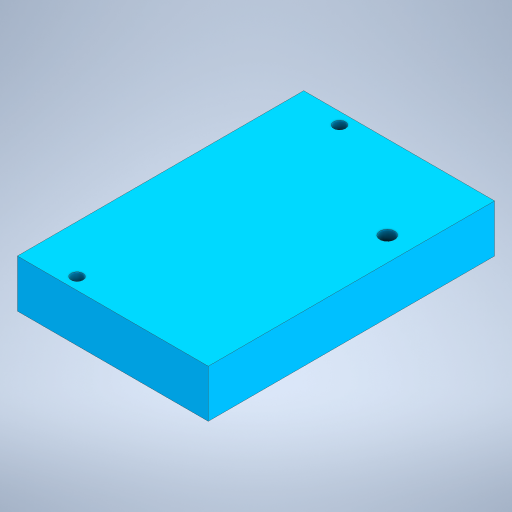
# Autodesk Inventor part: Top Plate for Side to Side motion
Saved by Autodesk Inventor 2023.1 (Build 271208000, 208)
## iProperties
Created: 2022-12-21
Part Number: Top Plate for Side to Side motion
Material: Generic
Document SubType Name: Modeling
Designer: shubh
Density: 1 g/cm^3
Appearance: Default
Author: shubh
Autodesk Inventor part; units mm, degrees
ref_plane "YZ Plane" through (0, 0, 0) normal (1, 0, 0) x (0, 1, 0)
ref_plane "XZ Plane" through (0, 0, 0) normal (0, 1, 0) x (-1, 0, 0)
ref_plane "XY Plane" through (0, 0, 0) normal (0, 0, 1) x (1, 0, 0)
sketch "Sketch1" plane through (0, 0, 0) normal (0, 1, 0) x (-1, 0, 0)
  line L0 (38.1, 76.2) -> (-63.5, 76.2)
  line L1 (-63.5, 76.2) -> (-63.5, -76.2)
  line L2 (-63.5, -76.2) -> (38.1, -76.2)
  line L3 (38.1, -76.2) -> (38.1, 76.2)
  circle A0 centre (-50.8, -31.75) radius 3.9751
  circle A1 centre (12.7, 69.85) radius 3.175
  circle A2 centre (12.7, -69.85) radius 3.175
  point P0 (0, 0)
  point P1 (38.1, 0)
  dimension "d0" = 152.4
  dimension "d1" = 101.6
  dimension "d2" = 38.1
  dimension "d6" = 7.9502
  dimension "d7" = 6.35
  dimension "d8" = 6.35
  dimension "d9" = 25.4
  dimension "d10" = 6.35
  dimension "d11" = 6.35
  dimension "d12" = 25.4
  dimension "d14" = 107.95
  dimension "d15" = 88.9
  constraints: 8 end point, 3 centre point, 2 parallel, 1 horizontal, 1 midpoint, 1 perpendicular
  measures "d0" distance of L2.end L0.start
  measures "d1" distance of L1.end L2.end
  measures "d2" distance from line of point (0, 0) L3
  measures "d6" diameter of A0
  measures "d7" diameter of A1
  measures "d8" distance from line of L0 A1.centre
  measures "d9" distance from line of L3 A1.centre
  measures "d10" diameter of A2
  measures "d11" distance from line of L2 A2.centre
  measures "d12" distance from line of L3 A2.centre
  measures "d14" distance from line of L0 A0.centre
  measures "d15" distance from line of L3 A0.centre
extrude "Extrusion1" add sketch "Sketch1" along normal blind 25.4
body "Solid1"
